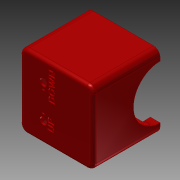
# Autodesk Inventor part: Durometer_Electronics_Enclosure_Lid
Saved by Autodesk Inventor 2015 (Build 190159000, 159)
## iProperties
Created: 2015-01-04
Part Number: Durometer_Electronics_Enclosure_Lid
Material: Generic
Document SubType Name: Modeling
Designer: Drew
Density: 1 g/cm^3
Appearance: Smooth - Red
Author: Drew
Autodesk Inventor part; units mm, degrees
ref_plane "YZ Plane" through (0, 0, 0) normal (1, 0, 0) x (0, 1, 0)
ref_plane "XZ Plane" through (0, 0, 0) normal (0, 1, 0) x (-1, 0, 0)
ref_plane "XY Plane" through (0, 0, 0) normal (0, 0, 1) x (1, 0, 0)
sketch "Sketch1" plane through (0, 0, 0) normal (0, 0, 1) x (1, 0, 0)
  line L0 (28.575, -34.925) -> (-28.575, -34.925)
  line L1 (-34.925, -28.575) -> (-34.925, 28.575)
  line L2 (-28.575, 34.925) -> (28.575, 34.925)
  line L3 (34.925, 28.575) -> (34.925, -28.575)
  line L4 (34.925, -34.925) -> (-34.925, 34.925) construction
  line L5 (-34.925, -34.925) -> (34.925, 34.925) construction
  arc A0 (-28.575, 34.925) -> (-34.925, 28.575) centre (-28.575, 28.575) ccw
  arc A1 (34.925, 28.575) -> (28.575, 34.925) centre (28.575, 28.575) ccw
  arc A2 (28.575, -34.925) -> (34.925, -28.575) centre (28.575, -28.575) ccw
  arc A3 (-34.925, -28.575) -> (-28.575, -34.925) centre (-28.575, -28.575) ccw
  point P0 (0, 0)
  dimension "d0" = 69.85
  dimension "d1" = 69.85
  dimension "d2" = 6.35
  constraints: 12 end point, 8 point on circle, 8 point on line, 8 tangent, 4 centre point, 3 equal radius, 2 midpoint, 2 parallel, 1 horizontal, 1 perpendicular
  measures "d0" distance of L4.end L5.end
  measures "d1" distance between parallel lines of L0 L2
  measures "d2" radius of A0
extrude "Extrusion1" add sketch "Sketch1" along normal blind 63.5
shell "Shell1" thickness 2.032 removed faces 1 at (9.525, 7.4083, 0)
sketch "Sketch4" plane through (0, 0, 0) normal (0, 0, -1) x (-1, 0, 0)
  arc A0 (-32.893, -28.575) -> (-28.575, -32.893) centre (-28.575, -28.575) ccw projected
  line L0 (-43.2886, 0) -> (36.2185, 0)
  line L1 (0, 45.1294) -> (0, -40.5019)
  line L2 (-28.575, -24.257) -> (-32.893, -24.257)
  line L3 (-24.257, -28.575) -> (-24.257, -32.893)
  line L4 (-24.257, -32.893) -> (-28.575, -32.893)
  line L5 (-32.893, -24.257) -> (-32.893, -28.575)
  arc A1 (-32.893, -28.575) -> (-28.575, -32.893) centre (-28.575, -28.575) ccw
  arc A2 (-24.257, -28.575) -> (-28.575, -24.257) centre (-28.575, -28.575) ccw
  arc A3 (-28.575, 32.893) -> (-32.893, 28.575) centre (-28.575, 28.575) ccw
  line L6 (-28.575, 24.257) -> (-32.893, 24.257)
  line L7 (-24.257, 28.575) -> (-24.257, 32.893)
  line L8 (-24.257, 32.893) -> (-28.575, 32.893)
  line L9 (-32.893, 24.257) -> (-32.893, 28.575)
  arc A4 (-28.575, 32.893) -> (-32.893, 28.575) centre (-28.575, 28.575) ccw
  arc A5 (-28.575, 24.257) -> (-24.257, 28.575) centre (-28.575, 28.575) ccw
  arc A6 (28.575, -32.893) -> (32.893, -28.575) centre (28.575, -28.575) ccw
  line L10 (28.575, -24.257) -> (32.893, -24.257)
  line L11 (24.257, -28.575) -> (24.257, -32.893)
  line L12 (24.257, -32.893) -> (28.575, -32.893)
  line L13 (32.893, -24.257) -> (32.893, -28.575)
  arc A7 (28.575, -32.893) -> (32.893, -28.575) centre (28.575, -28.575) ccw
  arc A8 (28.575, -24.257) -> (24.257, -28.575) centre (28.575, -28.575) ccw
  arc A9 (32.893, 28.575) -> (28.575, 32.893) centre (28.575, 28.575) ccw
  line L14 (28.575, 24.257) -> (32.893, 24.257)
  line L15 (24.257, 28.575) -> (24.257, 32.893)
  line L16 (24.257, 32.893) -> (28.575, 32.893)
  line L17 (32.893, 24.257) -> (32.893, 28.575)
  arc A10 (32.893, 28.575) -> (28.575, 32.893) centre (28.575, 28.575) ccw
  arc A11 (24.257, 28.575) -> (28.575, 24.257) centre (28.575, 28.575) ccw
  circle A12 centre (-28.575, -28.575) radius 1.45
  circle A13 centre (-28.575, 28.575) radius 1.45
  circle A14 centre (28.575, -28.575) radius 1.45
  circle A15 centre (28.575, 28.575) radius 1.45
  point P0 (0, 0)
  dimension "d7" = 4.318
  dimension "d8" = 4.318
  dimension "d11" = 2.9
  constraints: 36 end point, 27 symmetric about line, 22 point on circle, 15 centre point, 5 coincident, 4 tangent, 2 horizontal, 2 point on line, 1 vertical, 12 other
  measures "d7" distance of L2.end L5.end
  measures "d8" distance of L3.start L3.end
  measures "d11" diameter of A12
extrude "Extrusion2" add sketch "Sketch4" against normal up to surface (61.468 mm away)
fillet "Fillet2" radius 3.175 24 edges at (33.0651, 33.0651, 63.5) (0, 34.925, 63.5) (-33.0651, 33.0651, 63.5) (-34.925, 0, 63.5) (-33.0651, -33.0651, 63.5) (0, -34.925, 63.5) (33.0651, -33.0651, 63.5) (34.925, 0, 63.5) (32.893, 0, 61.468) (24.257, -30.734, 61.468) (30.734, -24.257, 61.468) (25.5217, -25.5217, 61.468) (0, -32.893, 61.468) (0, 32.893, 61.468) (30.734, 24.257, 61.468) (24.257, 30.734, 61.468) (25.5217, 25.5217, 61.468) (-30.734, -24.257, 61.468) (-24.257, -30.734, 61.468) (-25.5217, -25.5217, 61.468) (-32.893, 0, 61.468) (-24.257, 30.734, 61.468) (-30.734, 24.257, 61.468) (-25.5217, 25.5217, 61.468)
sketch "Sketch5" plane through (0, 0, 63.5) normal (0, 0, 1) x (1, 0, 0)
  circle A0 centre (-12.7, -15.875) radius 3.429
  line L0 (-50.1018, 0) -> (45.2159, 0)
  line L1 (-12.7, -24.1987) -> (-12.7, -7.4873)
  line L2 (-11.43, -9.144) -> (-13.97, -9.144)
  line L3 (-13.97, -9.144) -> (-13.97, -10.414)
  line L4 (-13.97, -10.414) -> (-11.43, -10.414)
  line L5 (-11.43, -10.414) -> (-11.43, -9.144)
  line L6 (-11.43, -9.144) -> (-13.97, -10.414) construction
  line L7 (-13.97, -9.144) -> (-11.43, -10.414) construction
  circle A1 centre (-12.7, 15.875) radius 3.429
  line L8 (-12.7, 24.1987) -> (-12.7, 7.4873)
  line L9 (-11.43, 9.144) -> (-13.97, 9.144)
  line L10 (-13.97, 9.144) -> (-13.97, 10.414)
  line L11 (-13.97, 10.414) -> (-11.43, 10.414)
  line L12 (-11.43, 10.414) -> (-11.43, 9.144)
  line L13 (-11.43, 9.144) -> (-13.97, 10.414) construction
  line L14 (-13.97, 9.144) -> (-11.43, 10.414) construction
  point P0 (0, 0)
  point P1 (-12.7, -9.779)
  point P2 (-12.7, 9.779)
  dimension "d31" = 6.096
  dimension "d32" = 6.858
  dimension "d33" = 2.54
  dimension "d34" = 1.27
  dimension "d35" = 31.75
  dimension "d36" = 12.7
  constraints: 30 end point, 8 symmetric about line, 4 midpoint, 3 point on line, 2 centre point, 2 horizontal, 2 parallel, 1 perpendicular, 1 vertical, 1 other
  measures "d31" distance of A0.centre point (-12.7, -9.779)
  measures "d32" diameter of A0
  measures "d33" distance of L2.start L2.end
  measures "d34" distance of L2.end L3.end
  measures "d35" diameter of A0.centre L0
  measures "d36" horizontal distance of point (0, 0) A0.centre
extrude "Extrusion3" cut sketch "Sketch5" against normal through all
sketch "Sketch6" plane through (0, 0, 63.5) normal (0, 0, 1) x (1, 0, 0)
  line L0 (-8.5246, -21.7298) -> (-8.5246, -16.5666) construction
  line L1 (-8.5246, -16.5666) -> (-5.3496, -16.5666) construction
  line L2 (-5.3496, -16.5666) -> (-5.3496, -21.7298) construction
  line L3 (-5.3496, -21.7298) -> (-8.5246, -21.7298) construction
  line L4 (-7.8723, 2.0585) -> (-7.8723, 14.6956) construction
  line L5 (-7.8723, 14.6956) -> (-4.6973, 14.6956) construction
  line L6 (-4.6973, 14.6956) -> (-4.6973, 2.0585) construction
  line L7 (-4.6973, 2.0585) -> (-7.8723, 2.0585) construction
  spline S0 degree 2 poles (-2.3002, -18.6324) (-2.3002, -19.8625) (-3.4858, -21.1864) (-4.6319, -21.1864) knots 0 0 0 1 2 2 2
  line L8 (-4.6319, -21.1864) -> (-8.5246, -21.1864)
  line L9 (-8.5246, -21.1864) -> (-8.5246, -19.655)
  line L10 (-8.5246, -19.655) -> (-4.7208, -19.655)
  spline S1 degree 2 poles (-4.7208, -19.655) (-4.0835, -19.655) (-3.4611, -19.1758) (-3.4611, -18.6324) knots 0 0 0 1 2 2 2
  spline S2 degree 2 poles (-3.4611, -18.6324) (-3.4611, -18.1038) (-4.0588, -17.6098) (-4.7208, -17.6098) knots 0 0 0 1 2 2 2
  line L11 (-4.7208, -17.6098) -> (-8.5246, -17.6098)
  line L12 (-8.5246, -17.6098) -> (-8.5246, -16.0784)
  line L13 (-8.5246, -16.0784) -> (-4.6368, -16.0784)
  spline S3 degree 2 poles (-4.6368, -16.0784) (-3.5105, -16.0784) (-2.3002, -17.3678) (-2.3002, -18.6324) knots 0 0 0 1 2 2 2
  spline S4 degree 2 poles (-6.6029, -10.2146) (-6.1781, -10.2146) (-5.4075, -10.4863) (-5.1506, -10.7382) knots 0 0 0 1 2 2 2
  spline S5 degree 2 poles (-5.1506, -10.7382) (-4.9876, -10.8914) (-4.7208, -11.2668) (-4.6269, -11.4891) knots 0 0 0 1 2 2 2
  spline S6 degree 2 poles (-4.6269, -11.4891) (-4.5331, -11.7164) (-4.4244, -12.2449) (-4.4244, -12.571) knots 0 0 0 1 2 2 2
  line L14 (-4.4244, -12.571) -> (-4.4244, -13.3713)
  line L15 (-4.4244, -13.3713) -> (-2.4286, -13.3713)
  line L16 (-2.4286, -13.3713) -> (-2.4286, -14.9027)
  line L17 (-2.4286, -14.9027) -> (-8.5246, -14.9027)
  line L18 (-8.5246, -14.9027) -> (-8.5246, -12.5364)
  spline S7 degree 2 poles (-8.5246, -12.5364) (-8.5246, -12.0128) (-8.332, -11.2471) (-8.1245, -10.9358) knots 0 0 0 1 2 2 2
  spline S8 degree 2 poles (-8.1245, -10.9358) (-7.8923, -10.59) (-7.1315, -10.2146) (-6.6029, -10.2146) knots 0 0 0 1 2 2 2
  spline S9 degree 2 poles (-6.5634, -11.7855) (-6.8252, -11.7855) (-7.1957, -12.0325) (-7.2649, -12.2005) knots 0 0 0 1 2 2 2
  spline S10 degree 2 poles (-7.2649, -12.2005) (-7.3588, -12.4178) (-7.3884, -12.813) (-7.3884, -13.1539) knots 0 0 0 1 2 2 2
  line L19 (-7.3884, -13.1539) -> (-7.3884, -13.3713)
  line L20 (-7.3884, -13.3713) -> (-5.5606, -13.3713)
  line L21 (-5.5606, -13.3713) -> (-5.5606, -13.2626)
  spline S11 degree 2 poles (-5.5606, -13.2626) (-5.5606, -13.0502) (-5.5705, -12.6648) (-5.5952, -12.5216) knots 0 0 0 1 2 2 2
  spline S12 degree 2 poles (-5.5952, -12.5216) (-5.6149, -12.3981) (-5.7335, -12.1264) (-5.8076, -12.0523) knots 0 0 0 1 2 2 2
  spline S13 degree 2 poles (-5.8076, -12.0523) (-5.9558, -11.8942) (-6.2868, -11.7855) (-6.5634, -11.7855) knots 0 0 0 1 2 2 2
  spline S14 degree 2 poles (-4.6909, 8.1298) (-3.8363, 8.1298) (-2.4926, 7.3839) (-2.132, 6.8158) knots 0 0 0 1 2 2 2
  spline S15 degree 2 poles (-2.132, 6.8158) (-1.8257, 6.3416) (-1.6479, 5.2251) (-1.6479, 4.5977) knots 0 0 0 1 2 2 2
  line L22 (-1.6479, 4.5977) -> (-1.6479, 2.6909)
  line L23 (-1.6479, 2.6909) -> (-7.7439, 2.6909)
  line L24 (-7.7439, 2.6909) -> (-7.7439, 4.578)
  spline S16 degree 2 poles (-7.7439, 4.578) (-7.7439, 5.2202) (-7.5809, 6.3416) (-7.2647, 6.8356) knots 0 0 0 1 2 2 2
  spline S17 degree 2 poles (-7.2647, 6.8356) (-6.8794, 7.4333) (-5.5752, 8.1298) (-4.6909, 8.1298) knots 0 0 0 1 2 2 2
  spline S18 degree 2 poles (-4.7008, 6.5589) (-5.3035, 6.5589) (-6.1631, 6.144) (-6.4051, 5.7191) knots 0 0 0 1 2 2 2
  spline S19 degree 2 poles (-6.4051, 5.7191) (-6.5731, 5.4079) (-6.6077, 4.7262) (-6.6077, 4.2519) knots 0 0 0 1 2 2 2
  line L25 (-6.6077, 4.2519) -> (-6.6077, 4.2223)
  line L26 (-6.6077, 4.2223) -> (-2.789, 4.2223)
  line L27 (-2.789, 4.2223) -> (-2.789, 4.2519)
  spline S20 degree 2 poles (-2.789, 4.2519) (-2.789, 4.7657) (-2.8236, 5.4721) (-3.0262, 5.7932) knots 0 0 0 1 2 2 2
  spline S21 degree 2 poles (-3.0262, 5.7932) (-3.2633, 6.1687) (-4.0981, 6.5589) (-4.7008, 6.5589) knots 0 0 0 1 2 2 2
  spline S22 degree 2 poles (-4.6959, 14.5865) (-3.2139, 14.5865) (-1.5194, 13.0057) (-1.5194, 11.6323) knots 0 0 0 1 2 2 2
  spline S23 degree 2 poles (-1.5194, 11.6323) (-1.5194, 10.2541) (-3.2336, 8.6831) (-4.6959, 8.6831) knots 0 0 0 1 2 2 2
  spline S24 degree 2 poles (-4.6959, 8.6831) (-6.1631, 8.6831) (-7.8723, 10.2541) (-7.8723, 11.6323) knots 0 0 0 1 2 2 2
  spline S25 degree 2 poles (-7.8723, 11.6323) (-7.8723, 13.0057) (-6.173, 14.5865) (-4.6959, 14.5865) knots 0 0 0 1 2 2 2
  spline S26 degree 2 poles (-4.6959, 13.0057) (-5.2442, 13.0057) (-6.0099, 12.7834) (-6.252, 12.5907) knots 0 0 0 1 2 2 2
  spline S27 degree 2 poles (-6.252, 12.5907) (-6.5039, 12.398) (-6.7213, 11.904) (-6.7213, 11.6373) knots 0 0 0 1 2 2 2
  spline S28 degree 2 poles (-6.7213, 11.6373) (-6.7213, 11.3557) (-6.5188, 10.8963) (-6.2619, 10.6838) knots 0 0 0 1 2 2 2
  spline S29 degree 2 poles (-6.2619, 10.6838) (-6.0248, 10.4961) (-5.2393, 10.2639) (-4.6959, 10.2639) knots 0 0 0 1 2 2 2
  spline S30 degree 2 poles (-4.6959, 10.2639) (-4.1327, 10.2639) (-3.3917, 10.4862) (-3.1398, 10.6789) knots 0 0 0 1 2 2 2
  spline S31 degree 2 poles (-3.1398, 10.6789) (-2.8878, 10.8716) (-2.6705, 11.3705) (-2.6705, 11.6373) knots 0 0 0 1 2 2 2
  spline S32 degree 2 poles (-2.6705, 11.6373) (-2.6705, 11.909) (-2.9027, 12.4129) (-3.1497, 12.5956) knots 0 0 0 1 2 2 2
  spline S33 degree 2 poles (-3.1497, 12.5956) (-3.4164, 12.7932) (-4.1228, 13.0057) (-4.6959, 13.0057) knots 0 0 0 1 2 2 2
  line L28 (-7.7439, 23.355) -> (-1.6479, 21.8137)
  line L29 (-1.6479, 21.8137) -> (-1.6479, 20.1341)
  line L30 (-1.6479, 20.1341) -> (-5.4171, 19.156)
  line L31 (-5.4171, 19.156) -> (-1.6479, 18.2125)
  line L32 (-1.6479, 18.2125) -> (-1.6479, 16.5279)
  line L33 (-1.6479, 16.5279) -> (-7.7439, 14.9866)
  line L34 (-7.7439, 14.9866) -> (-7.7439, 16.5773)
  line L35 (-7.7439, 16.5773) -> (-3.6634, 17.4171)
  line L36 (-3.6634, 17.4171) -> (-7.7439, 18.4348)
  line L37 (-7.7439, 18.4348) -> (-7.7439, 19.9563)
  line L38 (-7.7439, 19.9563) -> (-3.6585, 20.9245)
  line L39 (-3.6585, 20.9245) -> (-7.7439, 21.8039)
  line L40 (-7.7439, 21.8039) -> (-7.7439, 23.355)
  line L41 (-1.6479, 29.3325) -> (-1.6479, 27.8603)
  line L42 (-1.6479, 27.8603) -> (-5.8963, 25.5089)
  line L43 (-5.8963, 25.5089) -> (-1.6479, 25.5089)
  line L44 (-1.6479, 25.5089) -> (-1.6479, 24.1109)
  line L45 (-1.6479, 24.1109) -> (-7.7439, 24.1109)
  line L46 (-7.7439, 24.1109) -> (-7.7439, 25.9881)
  line L47 (-7.7439, 25.9881) -> (-4.2513, 27.9344)
  line L48 (-4.2513, 27.9344) -> (-7.7439, 27.9344)
  line L49 (-7.7439, 27.9344) -> (-7.7439, 29.3325)
  line L50 (-7.7439, 29.3325) -> (-1.6479, 29.3325)
  point P0 (0, 0)
  point P1 (-7.8723, 8.3771)
  point P2 (-8.5246, -19.1482)
  dimension "d39" = 3.175
  dimension "d40" = 3.175
  dimension "d41" = 5.1631
  dimension "d42" = 12.637
  constraints: 2 midpoint, 4 other
  measures "d39" distance of L2.end L0.start
  measures "d40" distance of L6.end L4.start
  measures "d41" distance of L1.end L2.end
  measures "d42" distance of L5.end L6.end
extrude "Extrusion4" cut sketch "Sketch6" against normal blind 1.27
sketch "Sketch7" plane through (34.925, -28.575, 0) normal (1, 0, 0) x (0, 0, -1)
  line L0 (-78.8961, 28.575) -> (28.5561, 28.575)
  arc A0 (0, 53.975) -> (0, 3.175) centre (0, 28.575) ccw
  line L1 (0, 3.175) -> (0, 53.975)
  line L2 (0, 4.318) -> (0, 52.832) projected
  point P0 (0, 28.575)
  dimension "d45" = 25.4
  constraints: 4 end point, 3 point on line, 2 point on circle, 1 centre point, 1 coincident, 1 horizontal, 1 midpoint
  measures "d45" radius of A0
extrude "Extrusion5" cut sketch "Sketch7" against normal up to next
equation "\"d1\" = d0"
equation "\"d8\" = d7"
equation "\"d40\" = d39"
body "Solid1"
